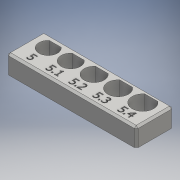
# Autodesk Inventor part: Fitting test
Saved by Autodesk Inventor 2016 (Build 200138000, 138)
## iProperties
Created: 2018-02-28
Part Number: Fitting test
Material: Generic
Document SubType Name: Modeling
Designer: Simon
Density: 1 g/cm^3
Appearance: Default
Author: Simon
Autodesk Inventor part; units mm, degrees
ref_plane "YZ Plane" through (0, 0, 0) normal (1, 0, 0) x (0, 1, 0)
ref_plane "XZ Plane" through (0, 0, 0) normal (0, 1, 0) x (-1, 0, 0)
ref_plane "XY Plane" through (0, 0, 0) normal (0, 0, 1) x (1, 0, 0)
sketch "Sketch1" plane through (0, 0, 0) normal (0, 0, 1) x (1, 0, 0)
  line L0 (0, 0) -> (35, 0)
  line L1 (35, 0) -> (35, 10)
  line L2 (35, 10) -> (0, 10)
  line L3 (0, 10) -> (0, 0)
  dimension "d3" = 35
  dimension "d4" = 10
  constraints: 8 end point, 2 parallel, 1 horizontal, 1 perpendicular
  measures "d3" distance of L2.end L1.end
  measures "d4" distance of L1.end L0.end
extrude "Extrusion1" add sketch "Sketch1" along normal blind 5
sketch "Sketch4" plane through (0, 0, 5) normal (0, 0, 1) x (1, 0, 0)
  line L0 (0, 10) -> (0, 0) projected
  arc A0 (2.8752, 8.6) -> (6.1248, 8.6) centre (4.5, 6.7) ccw
  line L1 (2.8752, 8.6) -> (6.1248, 8.6)
  line L2 (35, 10) -> (0, 10) projected
  line L3 (12.2613, 8.7) -> (8.9387, 8.7)
  arc A1 (8.9387, 8.7) -> (12.2613, 8.7) centre (10.6, 6.7) ccw
  line L4 (15.2029, 8.8) -> (18.5971, 8.8)
  arc A2 (15.2029, 8.8) -> (18.5971, 8.8) centre (16.9, 6.7) ccw
  line L5 (25.1321, 8.9) -> (21.6679, 8.9)
  arc A3 (21.6679, 8.9) -> (25.1321, 8.9) centre (23.4, 6.7) ccw
  line L6 (28.3336, 9) -> (31.8664, 9)
  arc A4 (28.3336, 9) -> (31.8664, 9) centre (30.1, 6.7) ccw
  dimension "d19" = 5
  dimension "d20" = 0.6
  dimension "d21" = 10
  dimension "d23" = 2
  dimension "d29" = 1
  dimension "d30" = 1
  dimension "d31" = 1
  dimension "d32" = 1
  dimension "d33" = 3.3
  constraints: 10 end point, 10 point on circle, 5 centre point, 4 horizontal alignment, 1 horizontal
  measures "d19" diameter of A0
  measures "d20" distance edge to line of A0 L1
  measures "d21" distance of L0.start L0.end
  measures "d23" distance edge to line of A0 L0
  measures "d33" distance from line of L2 A0.centre
extrude "Extrusion2" cut sketch "Sketch4" against normal through all
sketch "Sketch5" plane through (0, 0, 5) normal (0, 0, 1) x (1, 0, 0)
  line L0 (3.6775, 3.3406) -> (6.304, 3.3406) construction
  line L1 (6.304, 3.3406) -> (6.304, 1.3578) construction
  line L2 (6.304, 1.3578) -> (3.6775, 1.3578) construction
  line L3 (3.6775, 1.3578) -> (3.6775, 3.3406) construction
  line L4 (8.8209, 3.3406) -> (12.0803, 3.3406) construction
  line L5 (12.0803, 3.3406) -> (12.0803, 1.2121) construction
  line L6 (12.0803, 1.2121) -> (8.8209, 1.2121) construction
  line L7 (8.8209, 1.2121) -> (8.8209, 3.3406) construction
  line L8 (15.0947, 3.3406) -> (17.9707, 3.3406) construction
  line L9 (17.9707, 3.3406) -> (17.9707, 1.7774) construction
  line L10 (17.9707, 1.7774) -> (15.0947, 1.7774) construction
  line L11 (15.0947, 1.7774) -> (15.0947, 3.3406) construction
  line L12 (21.5368, 3.3406) -> (24.4128, 3.3406) construction
  line L13 (24.4128, 3.3406) -> (24.4128, 1.7774) construction
  line L14 (24.4128, 1.7774) -> (21.5368, 1.7774) construction
  line L15 (21.5368, 1.7774) -> (21.5368, 3.3406) construction
  line L16 (28.222, 3.3406) -> (34.9327, 3.3406) construction
  line L17 (34.9327, 3.3406) -> (34.9327, -0.2332) construction
  line L18 (34.9327, -0.2332) -> (28.222, -0.2332) construction
  line L19 (28.222, -0.2332) -> (28.222, 3.3406) construction
  spline S0 degree 2 poles (5.0357, 1.9759) (5.0357, 1.8316) (4.9433, 1.5853) (4.8591, 1.4945) knots 0 0 0 1 2 2 2
  spline S1 degree 2 poles (4.8591, 1.4945) (4.7748, 1.4038) (4.5236, 1.2984) (4.368, 1.2984) knots 0 0 0 1 2 2 2
  spline S2 degree 2 poles (4.368, 1.2984) (4.2253, 1.2984) (3.9466, 1.3616) (3.8445, 1.4119) knots 0 0 0 1 2 2 2
  line L20 (3.8445, 1.4119) -> (3.8445, 1.6955)
  line L21 (3.8445, 1.6955) -> (3.8639, 1.6955)
  spline S3 degree 2 poles (3.8639, 1.6955) (3.8947, 1.6728) (4.0098, 1.6145) (4.0795, 1.5885) knots 0 0 0 1 2 2 2
  spline S4 degree 2 poles (4.0795, 1.5885) (4.1589, 1.561) (4.2902, 1.5302) (4.3728, 1.5302) knots 0 0 0 1 2 2 2
  spline S5 degree 2 poles (4.3728, 1.5302) (4.4539, 1.5302) (4.6062, 1.5885) (4.6613, 1.6517) knots 0 0 0 1 2 2 2
  spline S6 degree 2 poles (4.6613, 1.6517) (4.7116, 1.7117) (4.7634, 1.8705) (4.7634, 1.9775) knots 0 0 0 1 2 2 2
  spline S7 degree 2 poles (4.7634, 1.9775) (4.7634, 2.0845) (4.7051, 2.2206) (4.65, 2.266) knots 0 0 0 1 2 2 2
  spline S8 degree 2 poles (4.65, 2.266) (4.5933, 2.3162) (4.4247, 2.3584) (4.3226, 2.3584) knots 0 0 0 1 2 2 2
  spline S9 degree 2 poles (4.3226, 2.3584) (4.2124, 2.3584) (3.9936, 2.3244) (3.9271, 2.3098) knots 0 0 0 1 2 2 2
  line L22 (3.9271, 2.3098) -> (3.9271, 3.3406)
  line L23 (3.9271, 3.3406) -> (5.0244, 3.3406)
  line L24 (5.0244, 3.3406) -> (5.0244, 3.1056)
  line L25 (5.0244, 3.1056) -> (4.1848, 3.1056)
  line L26 (4.1848, 3.1056) -> (4.1848, 2.5723)
  spline S10 degree 2 poles (4.1848, 2.5723) (4.2334, 2.5788) (4.3275, 2.5837) (4.3664, 2.5837) knots 0 0 0 1 2 2 2
  spline S11 degree 2 poles (4.3664, 2.5837) (4.5203, 2.5837) (4.7326, 2.5334) (4.8299, 2.4589) knots 0 0 0 1 2 2 2
  spline S12 degree 2 poles (4.8299, 2.4589) (4.9287, 2.3843) (5.0357, 2.1574) (5.0357, 1.9759) knots 0 0 0 1 2 2 2
  spline S13 degree 2 poles (10.179, 1.9694) (10.179, 1.8252) (10.0867, 1.5788) (10.0024, 1.488) knots 0 0 0 1 2 2 2
  spline S14 degree 2 poles (10.0024, 1.488) (9.9181, 1.3973) (9.6669, 1.2919) (9.5113, 1.2919) knots 0 0 0 1 2 2 2
  spline S15 degree 2 poles (9.5113, 1.2919) (9.3687, 1.2919) (9.0899, 1.3551) (8.9878, 1.4054) knots 0 0 0 1 2 2 2
  line L27 (8.9878, 1.4054) -> (8.9878, 1.689)
  line L28 (8.9878, 1.689) -> (9.0072, 1.689)
  spline S16 degree 2 poles (9.0072, 1.689) (9.038, 1.6663) (9.1531, 1.608) (9.2228, 1.5821) knots 0 0 0 1 2 2 2
  spline S17 degree 2 poles (9.2228, 1.5821) (9.3022, 1.5545) (9.4335, 1.5237) (9.5162, 1.5237) knots 0 0 0 1 2 2 2
  spline S18 degree 2 poles (9.5162, 1.5237) (9.5972, 1.5237) (9.7495, 1.5821) (9.8047, 1.6453) knots 0 0 0 1 2 2 2
  spline S19 degree 2 poles (9.8047, 1.6453) (9.8549, 1.7052) (9.9068, 1.8641) (9.9068, 1.971) knots 0 0 0 1 2 2 2
  spline S20 degree 2 poles (9.9068, 1.971) (9.9068, 2.078) (9.8484, 2.2141) (9.7933, 2.2595) knots 0 0 0 1 2 2 2
  spline S21 degree 2 poles (9.7933, 2.2595) (9.7366, 2.3098) (9.568, 2.3519) (9.4659, 2.3519) knots 0 0 0 1 2 2 2
  spline S22 degree 2 poles (9.4659, 2.3519) (9.3557, 2.3519) (9.1369, 2.3179) (9.0705, 2.3033) knots 0 0 0 1 2 2 2
  line L29 (9.0705, 2.3033) -> (9.0705, 3.3341)
  line L30 (9.0705, 3.3341) -> (10.1677, 3.3341)
  line L31 (10.1677, 3.3341) -> (10.1677, 3.0991)
  line L32 (10.1677, 3.0991) -> (9.3282, 3.0991)
  line L33 (9.3282, 3.0991) -> (9.3282, 2.5658)
  spline S23 degree 2 poles (9.3282, 2.5658) (9.3768, 2.5723) (9.4708, 2.5772) (9.5097, 2.5772) knots 0 0 0 1 2 2 2
  spline S24 degree 2 poles (9.5097, 2.5772) (9.6637, 2.5772) (9.876, 2.5269) (9.9732, 2.4524) knots 0 0 0 1 2 2 2
  spline S25 degree 2 poles (9.9732, 2.4524) (10.0721, 2.3778) (10.179, 2.1509) (10.179, 1.9694) knots 0 0 0 1 2 2 2
  line L34 (10.897, 1.3341) -> (10.5761, 1.3341)
  line L35 (10.5761, 1.3341) -> (10.5761, 1.7166)
  line L36 (10.5761, 1.7166) -> (10.897, 1.7166)
  line L37 (10.897, 1.7166) -> (10.897, 1.3341)
  line L38 (12.4335, 1.3341) -> (11.4578, 1.3341)
  line L39 (11.4578, 1.3341) -> (11.4578, 1.5383)
  line L40 (11.4578, 1.5383) -> (11.8209, 1.5383)
  line L41 (11.8209, 1.5383) -> (11.8209, 2.8786)
  line L42 (11.8209, 2.8786) -> (11.4578, 2.8786)
  line L43 (11.4578, 2.8786) -> (11.4578, 3.0618)
  spline S26 degree 2 poles (11.4578, 3.0618) (11.6637, 3.0618) (11.8581, 3.1785) (11.8711, 3.3406) knots 0 0 0 1 2 2 2
  line L44 (11.8711, 3.3406) -> (12.0786, 3.3406)
  line L45 (12.0786, 3.3406) -> (12.0786, 1.5383)
  line L46 (12.0786, 1.5383) -> (12.4335, 1.5383)
  line L47 (12.4335, 1.5383) -> (12.4335, 1.3341)
  spline S27 degree 2 poles (16.4529, 1.9338) (16.4529, 1.7895) (16.3605, 1.5432) (16.2762, 1.4524) knots 0 0 0 1 2 2 2
  spline S28 degree 2 poles (16.2762, 1.4524) (16.1919, 1.3616) (15.9407, 1.2563) (15.7851, 1.2563) knots 0 0 0 1 2 2 2
  spline S29 degree 2 poles (15.7851, 1.2563) (15.6425, 1.2563) (15.3637, 1.3195) (15.2616, 1.3697) knots 0 0 0 1 2 2 2
  line L48 (15.2616, 1.3697) -> (15.2616, 1.6534)
  line L49 (15.2616, 1.6534) -> (15.2811, 1.6534)
  spline S30 degree 2 poles (15.2811, 1.6534) (15.3119, 1.6307) (15.4269, 1.5723) (15.4966, 1.5464) knots 0 0 0 1 2 2 2
  spline S31 degree 2 poles (15.4966, 1.5464) (15.576, 1.5188) (15.7073, 1.488) (15.79, 1.488) knots 0 0 0 1 2 2 2
  spline S32 degree 2 poles (15.79, 1.488) (15.871, 1.488) (16.0234, 1.5464) (16.0785, 1.6096) knots 0 0 0 1 2 2 2
  spline S33 degree 2 poles (16.0785, 1.6096) (16.1287, 1.6696) (16.1806, 1.8284) (16.1806, 1.9354) knots 0 0 0 1 2 2 2
  spline S34 degree 2 poles (16.1806, 1.9354) (16.1806, 2.0423) (16.1222, 2.1785) (16.0671, 2.2239) knots 0 0 0 1 2 2 2
  spline S35 degree 2 poles (16.0671, 2.2239) (16.0104, 2.2741) (15.8418, 2.3162) (15.7397, 2.3162) knots 0 0 0 1 2 2 2
  spline S36 degree 2 poles (15.7397, 2.3162) (15.6295, 2.3162) (15.4107, 2.2822) (15.3443, 2.2676) knots 0 0 0 1 2 2 2
  line L50 (15.3443, 2.2676) -> (15.3443, 3.2984)
  line L51 (15.3443, 3.2984) -> (16.4415, 3.2984)
  line L52 (16.4415, 3.2984) -> (16.4415, 3.0634)
  line L53 (16.4415, 3.0634) -> (15.602, 3.0634)
  line L54 (15.602, 3.0634) -> (15.602, 2.5302)
  spline S37 degree 2 poles (15.602, 2.5302) (15.6506, 2.5367) (15.7446, 2.5415) (15.7835, 2.5415) knots 0 0 0 1 2 2 2
  spline S38 degree 2 poles (15.7835, 2.5415) (15.9375, 2.5415) (16.1498, 2.4913) (16.247, 2.4167) knots 0 0 0 1 2 2 2
  spline S39 degree 2 poles (16.247, 2.4167) (16.3459, 2.3422) (16.4529, 2.1153) (16.4529, 1.9338) knots 0 0 0 1 2 2 2
  line L55 (17.1709, 1.2984) -> (16.8499, 1.2984)
  line L56 (16.8499, 1.2984) -> (16.8499, 1.6809)
  line L57 (16.8499, 1.6809) -> (17.1709, 1.6809)
  line L58 (17.1709, 1.6809) -> (17.1709, 1.2984)
  line L59 (18.8078, 1.2984) -> (17.5744, 1.2984)
  line L60 (17.5744, 1.2984) -> (17.5744, 1.5821)
  spline S40 degree 2 poles (17.5744, 1.5821) (17.7073, 1.7068) (17.944, 1.9386) (18.0574, 2.0634) knots 0 0 0 1 2 2 2
  spline S41 degree 2 poles (18.0574, 2.0634) (18.2859, 2.3146) (18.4529, 2.6161) (18.4529, 2.7765) knots 0 0 0 1 2 2 2
  spline S42 degree 2 poles (18.4529, 2.7765) (18.4529, 2.8608) (18.401, 2.9872) (18.354, 3.0278) knots 0 0 0 1 2 2 2
  spline S43 degree 2 poles (18.354, 3.0278) (18.307, 3.0683) (18.1838, 3.1088) (18.1093, 3.1088) knots 0 0 0 1 2 2 2
  spline S44 degree 2 poles (18.1093, 3.1088) (18.038, 3.1088) (17.8921, 3.0731) (17.8256, 3.0456) knots 0 0 0 1 2 2 2
  spline S45 degree 2 poles (17.8256, 3.0456) (17.7689, 3.0229) (17.6636, 2.9581) (17.6311, 2.9354) knots 0 0 0 1 2 2 2
  line L61 (17.6311, 2.9354) -> (17.6166, 2.9354)
  line L62 (17.6166, 2.9354) -> (17.6166, 3.2206)
  spline S46 degree 2 poles (17.6166, 3.2206) (17.6992, 3.2611) (17.9958, 3.3406) (18.1287, 3.3406) knots 0 0 0 1 2 2 2
  spline S47 degree 2 poles (18.1287, 3.3406) (18.4091, 3.3406) (18.7252, 3.044) (18.7252, 2.7911) knots 0 0 0 1 2 2 2
  spline S48 degree 2 poles (18.7252, 2.7911) (18.7252, 2.6728) (18.67, 2.4751) (18.6214, 2.3908) knots 0 0 0 1 2 2 2
  spline S49 degree 2 poles (18.6214, 2.3908) (18.5728, 2.3033) (18.4318, 2.1315) (18.354, 2.0488) knots 0 0 0 1 2 2 2
  spline S50 degree 2 poles (18.354, 2.0488) (18.2276, 1.9111) (17.918, 1.6161) (17.8256, 1.5302) knots 0 0 0 1 2 2 2
  line L63 (17.8256, 1.5302) -> (18.8078, 1.5302)
  line L64 (18.8078, 1.5302) -> (18.8078, 1.2984)
  spline S51 degree 2 poles (22.895, 1.9338) (22.895, 1.7895) (22.8026, 1.5432) (22.7184, 1.4524) knots 0 0 0 1 2 2 2
  spline S52 degree 2 poles (22.7184, 1.4524) (22.6341, 1.3616) (22.3829, 1.2563) (22.2273, 1.2563) knots 0 0 0 1 2 2 2
  spline S53 degree 2 poles (22.2273, 1.2563) (22.0846, 1.2563) (21.8059, 1.3195) (21.7038, 1.3697) knots 0 0 0 1 2 2 2
  line L65 (21.7038, 1.3697) -> (21.7038, 1.6534)
  line L66 (21.7038, 1.6534) -> (21.7232, 1.6534)
  spline S54 degree 2 poles (21.7232, 1.6534) (21.754, 1.6307) (21.8691, 1.5723) (21.9388, 1.5464) knots 0 0 0 1 2 2 2
  spline S55 degree 2 poles (21.9388, 1.5464) (22.0182, 1.5188) (22.1495, 1.488) (22.2321, 1.488) knots 0 0 0 1 2 2 2
  spline S56 degree 2 poles (22.2321, 1.488) (22.3132, 1.488) (22.4655, 1.5464) (22.5206, 1.6096) knots 0 0 0 1 2 2 2
  spline S57 degree 2 poles (22.5206, 1.6096) (22.5709, 1.6696) (22.6227, 1.8284) (22.6227, 1.9354) knots 0 0 0 1 2 2 2
  spline S58 degree 2 poles (22.6227, 1.9354) (22.6227, 2.0423) (22.5644, 2.1785) (22.5093, 2.2239) knots 0 0 0 1 2 2 2
  spline S59 degree 2 poles (22.5093, 2.2239) (22.4526, 2.2741) (22.284, 2.3162) (22.1819, 2.3162) knots 0 0 0 1 2 2 2
  spline S60 degree 2 poles (22.1819, 2.3162) (22.0717, 2.3162) (21.8529, 2.2822) (21.7864, 2.2676) knots 0 0 0 1 2 2 2
  line L67 (21.7864, 2.2676) -> (21.7864, 3.2984)
  line L68 (21.7864, 3.2984) -> (22.8837, 3.2984)
  line L69 (22.8837, 3.2984) -> (22.8837, 3.0634)
  line L70 (22.8837, 3.0634) -> (22.0441, 3.0634)
  line L71 (22.0441, 3.0634) -> (22.0441, 2.5302)
  spline S61 degree 2 poles (22.0441, 2.5302) (22.0928, 2.5367) (22.1868, 2.5415) (22.2257, 2.5415) knots 0 0 0 1 2 2 2
  spline S62 degree 2 poles (22.2257, 2.5415) (22.3796, 2.5415) (22.5919, 2.4913) (22.6892, 2.4167) knots 0 0 0 1 2 2 2
  spline S63 degree 2 poles (22.6892, 2.4167) (22.7881, 2.3422) (22.895, 2.1153) (22.895, 1.9338) knots 0 0 0 1 2 2 2
  line L72 (23.613, 1.2984) -> (23.2921, 1.2984)
  line L73 (23.2921, 1.2984) -> (23.2921, 1.6809)
  line L74 (23.2921, 1.6809) -> (23.613, 1.6809)
  line L75 (23.613, 1.6809) -> (23.613, 1.2984)
  spline S64 degree 2 poles (24.5563, 3.1088) (24.4834, 3.1088) (24.3391, 3.0731) (24.2694, 3.0456) knots 0 0 0 1 2 2 2
  spline S65 degree 2 poles (24.2694, 3.0456) (24.2046, 3.018) (24.109, 2.9597) (24.0717, 2.9338) knots 0 0 0 1 2 2 2
  line L76 (24.0717, 2.9338) -> (24.0555, 2.9338)
  line L77 (24.0555, 2.9338) -> (24.0555, 3.2174)
  spline S66 degree 2 poles (24.0555, 3.2174) (24.143, 3.2644) (24.4428, 3.3406) (24.5774, 3.3406) knots 0 0 0 1 2 2 2
  spline S67 degree 2 poles (24.5774, 3.3406) (24.7135, 3.3406) (24.9161, 3.2855) (24.9987, 3.2271) knots 0 0 0 1 2 2 2
  spline S68 degree 2 poles (24.9987, 3.2271) (25.0863, 3.1639) (25.177, 2.9808) (25.177, 2.8576) knots 0 0 0 1 2 2 2
  spline S69 degree 2 poles (25.177, 2.8576) (25.177, 2.6923) (24.9599, 2.4427) (24.8075, 2.4103) knots 0 0 0 1 2 2 2
  line L78 (24.8075, 2.4103) -> (24.8075, 2.3908)
  spline S70 degree 2 poles (24.8075, 2.3908) (24.8707, 2.3778) (25.015, 2.3195) (25.0765, 2.2611) knots 0 0 0 1 2 2 2
  spline S71 degree 2 poles (25.0765, 2.2611) (25.1381, 2.2044) (25.2159, 2.0229) (25.2159, 1.8916) knots 0 0 0 1 2 2 2
  spline S72 degree 2 poles (25.2159, 1.8916) (25.2159, 1.7571) (25.1235, 1.5286) (25.0393, 1.441) knots 0 0 0 1 2 2 2
  spline S73 degree 2 poles (25.0393, 1.441) (24.9517, 1.3503) (24.7038, 1.2563) (24.5466, 1.2563) knots 0 0 0 1 2 2 2
  spline S74 degree 2 poles (24.5466, 1.2563) (24.3958, 1.2563) (24.1009, 1.3292) (24.0004, 1.3795) knots 0 0 0 1 2 2 2
  line L79 (24.0004, 1.3795) -> (24.0004, 1.6631)
  line L80 (24.0004, 1.6631) -> (24.0198, 1.6631)
  spline S75 degree 2 poles (24.0198, 1.6631) (24.1041, 1.6015) (24.3893, 1.488) (24.5304, 1.488) knots 0 0 0 1 2 2 2
  spline S76 degree 2 poles (24.5304, 1.488) (24.613, 1.488) (24.7783, 1.5399) (24.8334, 1.5999) knots 0 0 0 1 2 2 2
  spline S77 degree 2 poles (24.8334, 1.5999) (24.8869, 1.6598) (24.9436, 1.8025) (24.9436, 1.9111) knots 0 0 0 1 2 2 2
  spline S78 degree 2 poles (24.9436, 1.9111) (24.9436, 2.0197) (24.8804, 2.1607) (24.8237, 2.2012) knots 0 0 0 1 2 2 2
  spline S79 degree 2 poles (24.8237, 2.2012) (24.767, 2.2417) (24.613, 2.2725) (24.5222, 2.2725) knots 0 0 0 1 2 2 2
  line L81 (24.5222, 2.2725) -> (24.4088, 2.2725)
  line L82 (24.4088, 2.2725) -> (24.4088, 2.4945)
  line L83 (24.4088, 2.4945) -> (24.4979, 2.4945)
  spline S80 degree 2 poles (24.4979, 2.4945) (24.6778, 2.4945) (24.9047, 2.6663) (24.9047, 2.83) knots 0 0 0 1 2 2 2
  spline S81 degree 2 poles (24.9047, 2.83) (24.9047, 2.9062) (24.8464, 3.0148) (24.7994, 3.0472) knots 0 0 0 1 2 2 2
  spline S82 degree 2 poles (24.7994, 3.0472) (24.7492, 3.0812) (24.626, 3.1088) (24.5563, 3.1088) knots 0 0 0 1 2 2 2
  spline S83 degree 2 poles (29.5802, 1.9759) (29.5802, 1.8316) (29.4878, 1.5853) (29.4035, 1.4945) knots 0 0 0 1 2 2 2
  spline S84 degree 2 poles (29.4035, 1.4945) (29.3193, 1.4038) (29.068, 1.2984) (28.9124, 1.2984) knots 0 0 0 1 2 2 2
  spline S85 degree 2 poles (28.9124, 1.2984) (28.7698, 1.2984) (28.4911, 1.3616) (28.3889, 1.4119) knots 0 0 0 1 2 2 2
  line L84 (28.3889, 1.4119) -> (28.3889, 1.6955)
  line L85 (28.3889, 1.6955) -> (28.4084, 1.6955)
  spline S86 degree 2 poles (28.4084, 1.6955) (28.4392, 1.6728) (28.5543, 1.6145) (28.624, 1.5885) knots 0 0 0 1 2 2 2
  spline S87 degree 2 poles (28.624, 1.5885) (28.7034, 1.561) (28.8346, 1.5302) (28.9173, 1.5302) knots 0 0 0 1 2 2 2
  spline S88 degree 2 poles (28.9173, 1.5302) (28.9983, 1.5302) (29.1507, 1.5885) (29.2058, 1.6517) knots 0 0 0 1 2 2 2
  spline S89 degree 2 poles (29.2058, 1.6517) (29.256, 1.7117) (29.3079, 1.8705) (29.3079, 1.9775) knots 0 0 0 1 2 2 2
  spline S90 degree 2 poles (29.3079, 1.9775) (29.3079, 2.0845) (29.2496, 2.2206) (29.1945, 2.266) knots 0 0 0 1 2 2 2
  spline S91 degree 2 poles (29.1945, 2.266) (29.1377, 2.3162) (28.9692, 2.3584) (28.8671, 2.3584) knots 0 0 0 1 2 2 2
  spline S92 degree 2 poles (28.8671, 2.3584) (28.7569, 2.3584) (28.5381, 2.3244) (28.4716, 2.3098) knots 0 0 0 1 2 2 2
  line L86 (28.4716, 2.3098) -> (28.4716, 3.3406)
  line L87 (28.4716, 3.3406) -> (29.5688, 3.3406)
  line L88 (29.5688, 3.3406) -> (29.5688, 3.1056)
  line L89 (29.5688, 3.1056) -> (28.7293, 3.1056)
  line L90 (28.7293, 3.1056) -> (28.7293, 2.5723)
  spline S93 degree 2 poles (28.7293, 2.5723) (28.7779, 2.5788) (28.8719, 2.5837) (28.9108, 2.5837) knots 0 0 0 1 2 2 2
  spline S94 degree 2 poles (28.9108, 2.5837) (29.0648, 2.5837) (29.2771, 2.5334) (29.3744, 2.4589) knots 0 0 0 1 2 2 2
  spline S95 degree 2 poles (29.3744, 2.4589) (29.4732, 2.3843) (29.5802, 2.1574) (29.5802, 1.9759) knots 0 0 0 1 2 2 2
  line L91 (30.2982, 1.3406) -> (29.9773, 1.3406)
  line L92 (29.9773, 1.3406) -> (29.9773, 1.7231)
  line L93 (29.9773, 1.7231) -> (30.2982, 1.7231)
  line L94 (30.2982, 1.7231) -> (30.2982, 1.3406)
  line L95 (31.9886, 2.0278) -> (31.7504, 2.0278)
  line L96 (31.7504, 2.0278) -> (31.7504, 1.3406)
  line L97 (31.7504, 1.3406) -> (31.4927, 1.3406)
  line L98 (31.4927, 1.3406) -> (31.4927, 2.0278)
  line L99 (31.4927, 2.0278) -> (30.6094, 2.0278)
  line L100 (30.6094, 2.0278) -> (30.6094, 2.3098)
  line L101 (30.6094, 2.3098) -> (31.504, 3.3406)
  line L102 (31.504, 3.3406) -> (31.7504, 3.3406)
  line L103 (31.7504, 3.3406) -> (31.7504, 2.2433)
  line L104 (31.7504, 2.2433) -> (31.9886, 2.2433)
  line L105 (31.9886, 2.2433) -> (31.9886, 2.0278)
  line L106 (31.4927, 2.2433) -> (31.4927, 3.0245)
  line L107 (31.4927, 3.0245) -> (30.8201, 2.2433)
  line L108 (30.8201, 2.2433) -> (31.4927, 2.2433)
  point P0 (0, 0)
  constraints: 4 horizontal alignment, 10 other
extrude "Extrusion3" cut sketch "Sketch5" against normal blind 1.5
chamfer "Chamfer1" distance 0.5 angle 45 8 edges at (17.5, 10, 5) (35, 5, 5) (17.5, 0, 5) (0, 5, 5) (0, 0, 2.5) (0, 10, 2.5) (35, 0, 2.5) (35, 10, 2.5)
body "Solid1"
